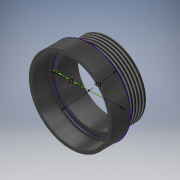
# Autodesk Inventor part: kaca lampu
Saved by Autodesk Inventor 2019.5 (Build 235369000, 369)
## iProperties
Created: 2022-10-10
Part Number: kaca lampu
Material: Aluminum 6061-AHC
Document SubType Name: Modeling
Designer: ASUS
Density: 2.7 g/cm^3
Appearance: Aluminum - Dark
Author: ASUS
Autodesk Inventor part; units mm, degrees
ref_plane "YZ Plane" through (0, 0, 0) normal (1, 0, 0) x (0, 1, 0)
ref_plane "XZ Plane" through (0, 0, 0) normal (0, 1, 0) x (-1, 0, 0)
ref_plane "XY Plane" through (0, 0, 0) normal (0, 0, 1) x (1, 0, 0)
sketch "Sketch1" plane through (0, 0, 0) normal (0, 0, 1) x (1, 0, 0)
  circle A0 centre (0, 0) radius 20
  circle A1 centre (0, 0) radius 18.5
  line L0 (-18.5, 0) -> (18.5, 0)
  circle A2 centre (0, 0) radius 17.5
  dimension "d8" = 40
  dimension "d9" = 35
  constraints: 3 centre point, 3 coincident, 2 end point, 2 point on circle, 1 horizontal
  measures "d8" diameter of A0
  measures "d9" diameter of A2
extrude "Extrusion1" add sketch "Sketch1" along normal blind 9
extrude "Extrusion2" add sketch "Sketch1" against normal blind 10 contours A2 L0 | L0 A2
sketch "Sketch2" plane through (0, 0, -10) normal (0, 0, -1) x (-1, 0, 0)
  point P0 (0, 0)
  point P1 (0, 0)
  constraints: 1 coincident
hole "Hole1" at (0, 0, -10) direction (0, 0, 1) diameter 31 depth 10.25
thread "Thread2" size "M35x1.5" class "6g" standard "ANSI Metric M Profile" full length
extrude "Extrusion3" add sketch "Sketch1" along normal blind 1 contours L0 A2 A1 | A1 L0 A2 | A2 L0 | L0 A2
sketch "Sketch3" plane through (0, 0, 0) normal (0, 0, -1) x (-1, 0, 0)
  point P0 (0, 0)
  point P1 (0, 0)
  constraints: 1 coincident
hole "Hole2" at (0, 0, 0) direction (0, 0, 1) diameter 35 depth 30
sketch "Sketch4" plane through (0, 0, 0) normal (1, 0, 0) x (0, 1, 0)
  point P0 (0, 0)
body "Solid1"
